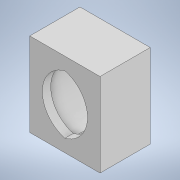
# Autodesk Inventor part: SpoolHolderJig
Saved by Autodesk Inventor 2021 (Build 250183000, 183)
## iProperties
Created: 2021-01-01
Part Number: SpoolHolderJig
Material: Generic
Document SubType Name: Modeling
Designer: elmar
Density: 1 g/cm^3
Appearance: Default
Author: elmar
Autodesk Inventor part; units mm, degrees
ref_plane "YZ Plane" through (0, 0, 0) normal (1, 0, 0) x (0, 1, 0)
ref_plane "XZ Plane" through (0, 0, 0) normal (0, 1, 0) x (-1, 0, 0)
ref_plane "XY Plane" through (0, 0, 0) normal (0, 0, 1) x (1, 0, 0)
sketch "Sketch1" plane through (0, 0, 0) normal (0, 0, 1) x (1, 0, 0)
  line L0 (0, -35) -> (0, 35) projected
  arc A0 (0, 19) -> (0, -19) centre (4.5333, 0) ccw
  arc A1 (0, -19) -> (0, 19) centre (-4.5333, 0) ccw
  line L1 (-29.4, 0) -> (29.4, 0) projected
  line L2 (21, -25) -> (-21, -25)
  line L3 (-21, -25) -> (-21, 25)
  line L4 (-21, 25) -> (21, 25)
  line L5 (21, 25) -> (21, -25)
  line L6 (21, -25) -> (-21, 25) construction
  line L7 (-21, -25) -> (21, 25) construction
  point P0 (0, 0)
  dimension "d0" = 38
  dimension "d1" = 30
  dimension "d2" = 6
  dimension "d3" = 6
  constraints: 12 end point, 4 point on circle, 3 point on line, 2 centre point, 2 midpoint, 2 parallel, 1 equal radius, 1 horizontal, 1 perpendicular
  measures "d0" distance of A0.end A0.start
  measures "d2" distance from line of A0.start L4
  measures "d3" distance edge to line of A1 L5
extrude "Extrusion1" add sketch "Sketch1" along normal blind 25 contours L2 L3 L1 A0 L0 | L0 A1 L1 L5 L2 | L1 L3 L4 L0 A0 | A1 L0 L4 L5 L1
sketch "Sketch2" plane through (0, 0, 25) normal (0, 0, 1) x (1, 0, 0)
  line L0 (-21, -25) -> (21, -25) projected
  line L1 (21, -25) -> (21, 25) projected
  line L2 (21, 25) -> (-21, 25) projected
  line L3 (-21, 25) -> (-21, -25) projected
  arc A0 (0, 19) -> (0, -19) centre (4.5333, 0) ccw projected
  arc A1 (0, -19) -> (0, 19) centre (-4.5333, 0) ccw projected
  arc A2 (0, 17.4542) -> (0, -17.4542) centre (4.5333, 0) ccw
  arc A3 (0, -17.4542) -> (0, 17.4542) centre (-4.5333, 0) ccw
  point P0 (0, 0)
  dimension "d11" = 1.5
  constraints: 4 point on circle, 2 centre point, 1 other
  measures "d11" radial gap between concentric circles of A1 A3
extrude "Extrusion2" add sketch "Sketch2" along normal blind 5 contours L3 L2 L1 L0 | A1 A0
thicken "Thicken2" operation add thickness 0.4 both sides no extend neighbours yes toward (0.9991799, -0.0404913, 0) faces at (14.984, -0.7909, 16.6667) (-14.6008, 3.9288, 16.6667)
body "Solid1"
